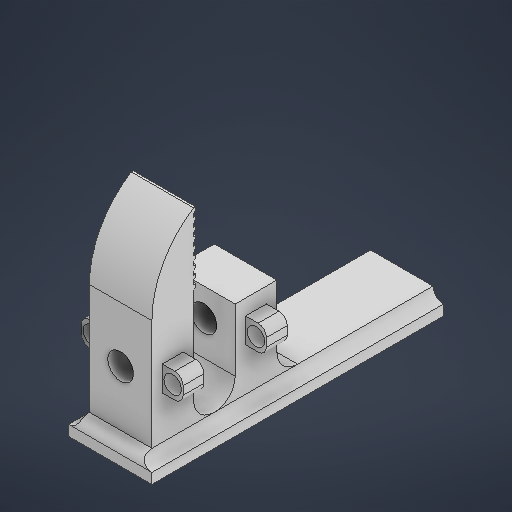
# Autodesk Inventor part: Garra
Saved by Autodesk Inventor 2026.1 (Build 301233020, 233B)
## iProperties
Created: 2025-11-06
Part Number: Garra
Material: Genérico
Document SubType Name: Modeling
Designer: luska
Density: 1 g/cm^3
Appearance: Padrão
Author: luska
Autodesk Inventor part; units mm, degrees
ref_plane "YZ Plane" through (0, 0, 0) normal (1, 0, 0) x (0, 1, 0)
ref_plane "XZ Plane" through (0, 0, 0) normal (0, 1, 0) x (-1, 0, 0)
ref_plane "XY Plane" through (0, 0, 0) normal (0, 0, 1) x (1, 0, 0)
sketch "Esboço1" plane through (0, 0, 0) normal (0, 1, 0) x (-1, 0, 0)
  point P0 (0, 0)
sketch "Esboço2" plane through (0, 0, 0) normal (0, 1, 0) x (-1, 0, 0)
  line L0 (18.622, 66.8641) -> (-1.378, 66.8641)
  line L1 (-1.378, 66.8641) -> (-1.378, -3.1359)
  line L2 (-1.378, -3.1359) -> (18.622, -3.1359)
  line L3 (18.622, -3.1359) -> (18.622, 66.8641)
  point P0 (0, 0)
  dimension "d0" = 70
  dimension "d1" = 20
  constraints: 8 end point, 2 parallel, 1 horizontal, 1 perpendicular
  measures "d0" distance between parallel lines of L2 L0
  measures "d1" distance between parallel lines of L3 L1
extrude "Extrusão1" add sketch "Esboço2" along normal blind 5
sketch "Esboço3" plane through (0, 5, 0) normal (0, 1, 0) x (1, 0, 0)
  line L0 (-1.122, -54.3641) -> (-16.122, -54.3641)
  line L1 (-16.122, -54.3641) -> (-16.122, -64.3641)
  line L2 (-16.122, -64.3641) -> (-1.122, -64.3641)
  line L3 (-1.122, -64.3641) -> (-1.122, -54.3641)
  line L4 (1.378, -66.8641) -> (1.378, 3.1359) projected
  line L5 (-18.622, -66.8641) -> (1.378, -66.8641) projected
  point P0 (0, 0)
  dimension "d4" = 10
  dimension "d5" = 15
  dimension "d6" = 2.5
  dimension "d11" = 2.5
  constraints: 8 end point, 2 parallel, 1 horizontal, 1 perpendicular
  measures "d4" distance between parallel lines of L2 L0
  measures "d5" distance between parallel lines of L1 L3
  measures "d6" distance between parallel lines of L4 L3
  measures "d11" distance between parallel lines of L5 L2
extrude "Extrusão2" add sketch "Esboço3" along normal blind 45
fillet "Arredondamento1" radius 2.5 2 edges at (-18.622, 5, 31.8641) (1.378, 5, 31.8641) inverted yes
fillet "Arredondamento2" radius 2.5 1 edges at (-8.622, 5, 66.8641)
sketch "Esboço4" plane through (-18.622, 0, -3.1359) normal (-1, 0, 0) x (0, 0, 1)
  point P0 (3.1359, 0)
sketch "Esboço5" plane through (0, 5, 0) normal (0, 1, 0) x (1, 0, 0)
  line L0 (-16.122, -34.3641) -> (-1.122, -34.3641)
  line L1 (-1.122, -34.3641) -> (-1.122, -44.3641)
  line L2 (-1.122, -44.3641) -> (-16.122, -44.3641)
  line L3 (-16.122, -44.3641) -> (-16.122, -34.3641)
  line L4 (-18.622, 3.1359) -> (-18.622, -66.8641) projected
  line L5 (-1.122, -54.3641) -> (-16.122, -54.3641) projected
  point P0 (0, 0)
  dimension "d12" = 15
  dimension "d13" = 10
  dimension "d14" = 2.5
  dimension "d15" = 10
  constraints: 8 end point, 2 parallel, 1 horizontal, 1 perpendicular
  measures "d12" distance of L1.end L2.end
  measures "d13" distance of L0.end L1.end
  measures "d14" distance between parallel lines of L4 L3
  measures "d15" distance between parallel lines of L5 L2
extrude "Extrusão3" add sketch "Esboço5" along normal blind 20
fillet "Arredondamento3" radius 22 1 edges at (-8.622, 50, 64.3641)
sketch "Esboço6" plane through (-1.122, 50, 54.3641) normal (0, 0, -1) x (-1, 0, 0)
  circle A0 centre (7.5, -31.71) radius 3.1
  line L0 (15, -41) -> (0, -41) projected
  line L1 (15, -45) -> (15, 0) projected
  line L2 (0, 0) -> (15, 0) projected
  point P0 (-1.122, -50)
  dimension "d20" = 6.2
  dimension "d22" = 7.5
  dimension "d34" = 31.71
  constraints: 1 centre point
  measures "d20" diameter of A0
  measures "d22" distance from line of L1 A0.centre
  measures "d34" distance from line of L2 A0.centre
extrude "Extrusão4" cut sketch "Esboço6" against normal blind 10
sketch "Esboço7" plane through (-1.122, 50, 54.3641) normal (0, 0, -1) x (-1, 0, 0)
  line L0 (10.7522, -36.7918) -> (4.7251, -37.0674)
  line L1 (4.7251, -37.0674) -> (1.4729, -31.9856)
  line L2 (1.4729, -31.9856) -> (4.2478, -26.6282)
  line L3 (4.2478, -26.6282) -> (10.2749, -26.3526)
  line L4 (10.2749, -26.3526) -> (13.5271, -31.4344)
  line L5 (13.5271, -31.4344) -> (10.7522, -36.7918)
  line L6 (15, -41) -> (0, -41) projected
  line L7 (15, -45) -> (15, 0) projected
  line L8 (0, 0) -> (15, 0) projected
  point P0 (-1.122, -50)
  point P1 (7.5, -31.71)
  dimension "d26" = 7.5
  dimension "d35" = 31.71
  constraints: 12 end point, 13 other
  measures "d26" distance from line of L7 point (7.5, -31.71)
  measures "d35" distance from line of L8 point (7.5, -31.71)
extrude "Extrusão5" cut sketch "Esboço7" against normal blind 5
sketch "Esboço8" plane through (-1.122, 25, 34.3641) normal (0, 0, -1) x (-1, 0, 0)
  circle A0 centre (7.5, -6.72) radius 3.1
  line L0 (0, 0) -> (15, 0) projected
  line L1 (0, -20) -> (0, 0) projected
  line L2 (0, -20) -> (15, -20) projected
  point P0 (-1.122, -25)
  point P1 (0, -16)
  point P2 (7.5, 0)
  dimension "d29" = 6.2
  dimension "d31" = 7.5
  dimension "d86" = 13.28
  constraints: 1 centre point, 1 midpoint
  measures "d29" diameter of A0
  measures "d31" distance from line of L1 A0.centre
  measures "d86" distance from line of L2 A0.centre
extrude "Extrusão6" cut sketch "Esboço8" against normal blind 10
sketch "Esboço10" plane through (-16.122, 5, 64.3641) normal (-1, 0, 0) x (0, 0, 1)
  line L0 (-22.5, 10.28) -> (-27.5, 10.28)
  line L1 (-27.5, 10.28) -> (-27.5, 16.28)
  line L2 (-27.5, 16.28) -> (-22.5, 16.28)
  line L3 (-22.5, 16.28) -> (-22.5, 10.28)
  line L4 (-30, 20) -> (-20, 20) projected
  line L5 (-20, 0) -> (-20, 20) projected
  line L6 (-20, 0) -> (-30, 0) projected
  line L7 (-3.0499, 10.28) -> (-8.0499, 10.28)
  line L8 (-8.0499, 10.28) -> (-8.0499, 16.28)
  line L9 (-8.0499, 16.28) -> (-3.0499, 16.28)
  line L10 (-3.0499, 16.28) -> (-3.0499, 10.28)
  line L11 (0, 0) -> (-10, 0) projected
  point P0 (-64.3641, -5)
  point P1 (-25, 16.28)
  point P2 (-20, 4)
  point P3 (-16, 0)
  point P4 (-34, 0)
  point P5 (-3.0499, 13.28)
  point P6 (-5.5499, 10.28)
  point P7 (-5.5499, 16.28)
  point P8 (-14, 0)
  dimension "d40" = 3.72
  dimension "d41" = 6
  dimension "d42" = 5
  dimension "d43" = 2.5
  dimension "d44" = 10.28
  dimension "d45" = 5
  dimension "d46" = 6
  dimension "d47" = 10.28
  constraints: 16 end point, 4 midpoint, 4 parallel, 2 horizontal, 2 perpendicular
  measures "d40" distance from line of L4 point (-25, 16.28)
  measures "d41" distance between parallel lines of L2 L0
  measures "d42" distance between parallel lines of L1 L3
  measures "d43" distance between parallel lines of L5 L3
  measures "d44" distance between parallel lines of L6 L0
  measures "d45" distance from line of L8 point (-3.05, 13.28)
  measures "d46" distance of point (-5.55, 10.28) point (-5.55, 16.28)
  measures "d47" distance between parallel lines of L11 L7
extrude "Extrusão8" add sketch "Esboço10" along normal blind 5
fillet "Arredondamento5" radius 2 4 edges at (-21.122, 15.28, 58.8142) (-21.122, 21.28, 58.8142) (-21.122, 21.28, 39.3641) (-21.122, 15.28, 39.3641)
sketch "Esboço11" plane through (-16.122, 15.28, 36.8641) normal (0, 0, -1) x (-1, 0, 0)
  circle A0 centre (2.5, 3) radius 2.1
  line L0 (5, 4) -> (5, 2) projected
  line L1 (0, 0) -> (3, 0) projected
  point P0 (-16.122, -15.28)
  point P1 (5, 3)
  dimension "d51" = 4.2
  dimension "d52" = 2.5
  dimension "d53" = 3
  constraints: 1 centre point, 1 midpoint
  measures "d51" diameter of A0
  measures "d52" distance of point (5, 3) A0.centre
  measures "d53" distance from line of L1 A0.centre
sketch "Esboço12" plane through (-16.122, 15.28, 56.3142) normal (0, 0, -1) x (-1, 0, 0)
  circle A0 centre (2.5, 3) radius 2.1
  line L0 (0, 0) -> (3, 0) projected
  line L1 (5, 4) -> (5, 2) projected
  point P0 (-16.122, -15.28)
  dimension "d54" = 4.2
  dimension "d55" = 3
  dimension "d56" = 2.5
  constraints: 1 centre point
  measures "d54" diameter of A0
  measures "d55" distance from line of L0 A0.centre
  measures "d56" distance from line of L1 A0.centre
sketch "Esboço13" plane through (-1.122, 25, 44.3641) normal (1, 0, 0) x (0, 0, -1)
  point P0 (44.3641, -25)
sketch "Esboço14" plane through (-1.122, 25, 44.3641) normal (1, 0, 0) x (0, 0, -1)
  line L0 (7.5, -9.72) -> (2.5, -9.72)
  line L1 (2.5, -9.72) -> (2.5, -3.72)
  line L2 (2.5, -3.72) -> (7.5, -3.72)
  line L3 (7.5, -3.72) -> (7.5, -9.72)
  line L4 (0, -20) -> (10, -20) projected
  point P0 (44.3641, -25)
  point P1 (5, -26.56)
  point P2 (2.5, -6.72)
  point P3 (-4, -20)
  point P4 (14, -20)
  dimension "d58" = 6
  dimension "d59" = 5
  dimension "d85" = 10.28
  constraints: 8 end point, 2 parallel, 1 horizontal, 1 midpoint, 1 perpendicular
  measures "d58" distance between parallel lines of L0 L2
  measures "d59" distance from line of point (2.5, -6.72) L3
  measures "d85" distance between parallel lines of L0 L4
sketch "Esboço15" plane through (-1.122, 5, 64.3641) normal (1, 0, 0) x (0, 0, -1)
  point P0 (64.3641, -5)
sketch "Esboço16" plane through (-1.122, 5, 64.3641) normal (1, 0, 0) x (0, 0, -1)
  point P0 (64.3641, -5)
extrude "Extrusão9" add sketch "Esboço14" along normal blind 5
extrude "Extrusão10" cut sketch "Esboço11" against normal blind 5
extrude "Extrusão11" cut sketch "Esboço12" against normal blind 5
sketch "Esboço17" plane through (-1.122, 5, 64.3641) normal (1, 0, 0) x (0, 0, -1)
  line L0 (2.5, 10.28) -> (7.5, 10.28)
  line L1 (7.5, 10.28) -> (7.5, 16.28)
  line L2 (7.5, 16.28) -> (2.5, 16.28)
  line L3 (2.5, 16.28) -> (2.5, 10.28)
  line L4 (10, 0) -> (10, 45) projected
  line L5 (10, 0) -> (0, 0) projected
  point P0 (64.3641, -5)
  point P1 (5, 10.28)
  point P2 (10, 4)
  point P3 (14, 0)
  dimension "d67" = 6
  dimension "d68" = 5
  dimension "d69" = 2.5
  dimension "d70" = 10.28
  constraints: 8 end point, 2 parallel, 1 horizontal, 1 midpoint, 1 perpendicular
  measures "d67" distance from line of point (5, 10.28) L2
  measures "d68" distance between parallel lines of L1 L3
  measures "d69" distance between parallel lines of L1 L4
  measures "d70" distance between parallel lines of L5 L0
extrude "Extrusão12" add sketch "Esboço17" along normal blind 5
sketch "Esboço18" plane through (-1.122, 15.28, 36.8641) normal (0, 0, -1) x (-1, 0, 0)
  circle A0 centre (-2.5, 3) radius 2.1
  point P0 (-1.122, -15.28)
  dimension "d73" = 4.2
  constraints: 1 centre point
  measures "d73" diameter of A0
sketch "Esboço19" plane through (-1.122, 15.28, 56.8641) normal (0, 0, -1) x (-1, 0, 0)
  circle A0 centre (-2.5, 3) radius 2.1
  point P0 (-1.122, -15.28)
  point P1 (-5, 3)
  dimension "d76" = 4.2
  dimension "d78" = 2.5
  constraints: 1 centre point
  measures "d76" diameter of A0
  measures "d78" distance of point (-5, 3) A0.centre
extrude "Extrusão13" cut sketch "Esboço18" against normal blind 5
extrude "Extrusão14" cut sketch "Esboço19" against normal blind 5
fillet "Arredondamento6" radius 2 4 edges at (3.878, 21.28, 39.3641) (3.878, 15.28, 39.3641) (3.878, 15.28, 59.3641) (3.878, 21.28, 59.3641)
sketch "Esboço20" plane through (-1.122, 25, 34.3641) normal (0, 0, -1) x (-1, 0, 0)
  point P0 (-1.122, -25)
sketch "Esboço21" plane through (-1.122, 5, 34.3641) normal (0, 0, -1) x (-1, 0, 0)
  line L0 (9.8438, 9.1967) -> (5.1356, 9.2086)
  line L1 (5.1356, 9.2086) -> (2.7918, 13.2919)
  line L2 (2.7918, 13.2919) -> (5.1562, 17.3633)
  line L3 (5.1562, 17.3633) -> (9.8644, 17.3514)
  line L4 (9.8644, 17.3514) -> (12.2082, 13.2681)
  line L5 (12.2082, 13.2681) -> (9.8438, 9.1967)
  line L6 (0, 0) -> (15, 0) projected
  line L7 (15, 0) -> (15, 20) projected
  point P0 (-1.122, -5)
  point P1 (7.5, 13.28)
  point P2 (7.5, 0)
  dimension "d87" = 13.28
  dimension "d88" = 7.5
  constraints: 12 end point, 1 midpoint, 13 other
  measures "d87" distance of point (7.5, 0) point (7.5, 13.28)
  measures "d88" distance from line of L7 point (7.5, 13.28)
extrude "Extrusão15" cut sketch "Esboço21" against normal blind 5
fillet "Arredondamento7" radius 5 3 edges at (-8.622, 5, 54.3641) (-8.622, 5, 34.3641) (-8.622, 5, 44.3641)
sketch "Esboço22" plane through (-1.122, 50, 54.3641) normal (0, 0, -1) x (-1, 0, 0)
  line L0 (15, 0) -> (15, -18.4391) projected
  line L1 (0, -18.4391) -> (0, 0) projected
  line L2 (15, 0) -> (0, 0)
  line L3 (0, 0) -> (0, -1)
  line L4 (0, -1) -> (15, -1)
  line L5 (15, -1) -> (15, 0)
  line L6 (7.8898, -1) -> (7.8898, -2.2265)
  line L7 (15, -1) -> (0, -1)
  line L8 (0, -1) -> (0, -2)
  line L9 (0, -2) -> (15, -2)
  line L10 (15, -2) -> (15, -1)
  line L11 (15, -2) -> (0, -2)
  line L12 (0, -2) -> (0, -3)
  line L13 (0, -3) -> (15, -3)
  line L14 (15, -3) -> (15, -2)
  line L15 (15, -3) -> (0, -3)
  line L16 (0, -3) -> (0, -4)
  line L17 (0, -4) -> (15, -4)
  line L18 (15, -4) -> (15, -3)
  line L19 (15, -4) -> (0, -4)
  line L20 (0, -4) -> (0, -5)
  line L21 (0, -5) -> (15, -5)
  line L22 (15, -5) -> (15, -4)
  line L23 (15, -5) -> (0, -5)
  line L24 (0, -5) -> (0, -6)
  line L25 (0, -6) -> (15, -6)
  line L26 (15, -6) -> (15, -5)
  line L27 (15, -6) -> (0, -6)
  line L28 (0, -6) -> (0, -7)
  line L29 (0, -7) -> (15, -7)
  line L30 (15, -7) -> (15, -6)
  line L31 (15, -7) -> (0, -7)
  line L32 (0, -7) -> (0, -8)
  line L33 (0, -8) -> (15, -8)
  line L34 (15, -8) -> (15, -7)
  line L35 (15, -8) -> (0, -8)
  line L36 (0, -8) -> (0, -9)
  line L37 (0, -9) -> (15, -9)
  line L38 (15, -9) -> (15, -8)
  line L39 (15, -9) -> (0, -9)
  line L40 (0, -9) -> (0, -10)
  line L41 (0, -10) -> (15, -10)
  line L42 (15, -10) -> (15, -9)
  line L43 (15, -10) -> (0, -10)
  line L44 (0, -10) -> (0, -11)
  line L45 (0, -11) -> (15, -11)
  line L46 (15, -11) -> (15, -10)
  line L47 (15, -11) -> (0, -11)
  line L48 (0, -11) -> (0, -12)
  line L49 (0, -12) -> (15, -12)
  line L50 (15, -12) -> (15, -11)
  line L51 (15, -12) -> (0, -12)
  line L52 (0, -12) -> (0, -13)
  line L53 (0, -13) -> (15, -13)
  line L54 (15, -13) -> (15, -12)
  line L55 (15, -13) -> (0, -13)
  line L56 (0, -13) -> (0, -14)
  line L57 (0, -14) -> (15, -14)
  line L58 (15, -14) -> (15, -13)
  line L59 (15, -14) -> (0, -14)
  line L60 (0, -14) -> (0, -15)
  line L61 (0, -15) -> (15, -15)
  line L62 (15, -15) -> (15, -14)
  line L63 (15, -15) -> (0, -15)
  line L64 (0, -15) -> (0, -16)
  line L65 (0, -16) -> (15, -16)
  line L66 (15, -16) -> (15, -15)
  line L67 (15, -16) -> (0, -16)
  line L68 (0, -16) -> (0, -17)
  line L69 (0, -17) -> (15, -17)
  line L70 (15, -17) -> (15, -16)
  point P0 (-1.122, -50)
  point P1 (7.8898, -2)
  point P2 (7.8898, -3)
  point P3 (7.8898, -4)
  point P4 (7.8898, -5)
  point P5 (7.8898, -6)
  point P6 (7.8898, -7)
  point P7 (7.8898, -8)
  point P8 (7.8898, -9)
  point P9 (7.8898, -10)
  point P10 (7.8898, -11)
  point P11 (7.8898, -12)
  point P12 (7.8898, -13)
  point P13 (7.8898, -14)
  point P14 (7.8898, -15)
  point P15 (7.8898, -16)
  point P16 (7.8898, -17)
  point P17 (0, -17)
  point P18 (0, -16)
  point P19 (0, -15)
  point P20 (15, -15)
  point P21 (0, -14)
  point P22 (0, -13)
  point P23 (0, -12)
  point P24 (0, -11)
  point P25 (15, -11)
  point P26 (15, -10)
  point P27 (0, -10)
  point P28 (0, -9)
  point P29 (15, -9)
  point P30 (15, -8)
  point P31 (0, -8)
  point P32 (0, -7)
  point P33 (15, -7)
  point P34 (15, -6)
  point P35 (0, -6)
  point P36 (0, -5)
  point P37 (15, -5)
  point P38 (15, -4)
  point P39 (0, -4)
  point P40 (0, -3)
  point P41 (15, -3)
  point P42 (15, -2)
  point P43 (0, -2)
  point P44 (15, -1)
  dimension "d92" = 1
  dimension "d95" = 1
  constraints: 138 end point, 17 point on line, 2 parallel, 2 vertical, 1 horizontal, 1 perpendicular, 146 other
  measures "d92" distance between parallel lines of L4 L2
  measures "d95" distance of L3.end L8.end
extrude "Extrusão16" add sketch "Esboço22" along normal blind 0.5 contours L0 L4 L1 L2 | L0 L13 L1 L9 | L0 L21 L1 L17 | L0 L29 L1 L25 | L0 L37 L1 L33 | L0 L45 L1 L41 | L0 L53 L1 L49 | L0 L61 L1 L57 | L0 L69 L1 L65
fillet "Arredondamento8" radius 0.7 9 edges at (-8.622, 33, 53.8641) (-8.622, 35, 53.8641) (-8.622, 37, 53.8641) (-8.622, 39, 53.8641) (-8.622, 41, 53.8641) (-8.622, 43, 53.8641) (-8.622, 45, 53.8641) (-8.622, 47, 53.8641) (-8.622, 49, 53.8641)
sketch "Esboço23" plane through (1.378, 0, -3.1359) normal (0, 0, -1) x (-1, 0, 0)
  point P0 (1.378, 0)
sketch "Esboço24" plane through (1.378, 0, -3.1359) normal (0, 0, -1) x (-1, 0, 0)
  point P0 (1.378, 0)
